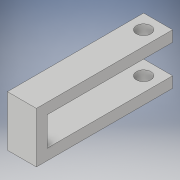
# Autodesk Inventor part: TensionerAxleHolder
Saved by Autodesk Inventor 2017 (Build 210142000, 142)
## iProperties
Created: 2017-07-29
Part Number: TensionerAxleHolder
Material: Generic
Document SubType Name: Modeling
Designer: User
Density: 1 g/cm^3
Appearance: Default
Author: User
Autodesk Inventor part; units mm, degrees
ref_plane "YZ Plane" through (0, 0, 0) normal (1, 0, 0) x (0, 1, 0)
ref_plane "XZ Plane" through (0, 0, 0) normal (0, 1, 0) x (-1, 0, 0)
ref_plane "XY Plane" through (0, 0, 0) normal (0, 0, 1) x (1, 0, 0)
sketch "Sketch1" plane through (0, 0, 0) normal (1, 0, 0) x (0, 1, 0)
  line L0 (0, 0) -> (22.225, 0)
  line L1 (22.225, 0) -> (22.225, -59.69)
  line L2 (0, -59.69) -> (0, 0)
  line L3 (4.7625, -59.69) -> (5.9323, -59.69)
  line L4 (4.7625, -59.69) -> (4.7625, -4.7625)
  line L5 (4.7625, -4.7625) -> (17.4625, -4.7625)
  line L6 (17.4625, -4.7625) -> (17.4625, -59.69)
  line L7 (22.225, -59.69) -> (17.4625, -59.69)
  line L8 (4.7625, -59.69) -> (0, -59.69)
  dimension "d1" = 59.69
  dimension "d4" = 12.7
  dimension "d6" = 4.7625
  dimension "d15" = 59.69
  dimension "d22" = 4.7625
  dimension "d24" = 4.7625
  constraints: 18 end point, 4 parallel, 2 horizontal, 1 perpendicular
  measures "d1" distance of L0.end L1.end
  measures "d4" distance of L4.end L5.end
  measures "d6" distance between parallel lines of L2 L4
  measures "d15" distance of L2.start L0.start
  measures "d22" distance between parallel lines of L1 L6
  measures "d24" distance between parallel lines of L0 L5
extrude "Extrusion1" add sketch "Sketch1" along normal blind 12.7
sketch "Sketch2" plane through (0, 22.225, 0) normal (0, 1, 0) x (1, 0, 0)
  circle A0 centre (6.35, 53.34) radius 3.175
  line L0 (0, 0) -> (0, 59.69) projected
  line L1 (0, 0) -> (12.7, 0) projected
  line L2 (12.7, 59.69) -> (12.7, 0) projected
  line L3 (0, 59.69) -> (12.7, 59.69) projected
  point P0 (0, 0)
  dimension "d9" = 6.35
  dimension "d10" = 12.7
  dimension "d11" = 6.35
  dimension "d16" = 6.35
  constraints: 1 centre point
  measures "d9" diameter of A0
  measures "d10" distance of L0.end L2.start
  measures "d11" distance from line of L0 A0.centre
  measures "d16" distance from line of L3 A0.centre
extrude "Extrusion2" cut sketch "Sketch2" against normal blind 25.4 contours A0
sketch "Sketch3" plane through (0, 4.7625, -4.7625) normal (0, 0, -1) x (-1, 0, 0)
  line L0 (0, 12.7) -> (0, 0) projected
  line L1 (0, 12.7) -> (-12.7, 12.7) projected
  line L2 (-12.7, 0) -> (-12.7, 12.7) projected
  line L3 (0, 0) -> (-12.7, 0) projected
  line L4 (0, 0) -> (-12.7, 0) projected
  line L5 (0, 0) -> (0, -4.7625) projected
  line L6 (0, 0) -> (-12.7, 0) projected
  line L7 (-12.7, -4.7625) -> (-12.7, 0) projected
  line L8 (0, -4.7625) -> (-12.7, -4.7625) projected
  circle A0 centre (-6.35, 6.35) radius 4.7625
  point P0 (0, -4.7625)
  dimension "d17" = 9.525
  dimension "d18" = 6.35
  dimension "d19" = 6.35
  dimension "d23" = 12.7
  constraints: 1 centre point
  measures "d17" diameter of A0
  measures "d18" distance from line of L0 A0.centre
  measures "d19" distance from line of L1 A0.centre
  measures "d23" distance of L5.end L7.start
extrude "Extrusion3" cut sketch "Sketch3" against normal blind 3.175 contours A0
equation "\"d15\" = d1"
equation "\"d11\" = 0.5 * d10"
equation "\"d16\" = d11"
equation "\"d18\" = 0.5 * d23"
body "Solid1"
